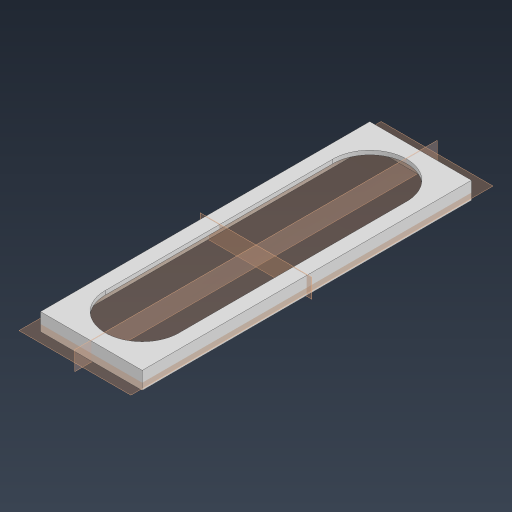
# Autodesk Inventor part: Крышка_крепления_динамика
Saved by Autodesk Inventor 2023.2 (Build 272271030, 271C)
## iProperties
Created: 2025-09-17
Part Number: Крышка_крепления_динамика
Material: Типовые
Document SubType Name: Modeling
Designer: Олег Коноваленко
Density: 1 g/cm^3
Appearance: По умолчанию
Author: Олег Коноваленко
Autodesk Inventor part; units mm, degrees
sketch "Эскиз1" plane through (0, 0, 0) normal (0, 1, 0) x (-1, 0, 0)
  line L0 (35, 120) -> (-35, 120)
  line L1 (-35, 120) -> (-35, -120)
  line L2 (-35, -120) -> (35, -120)
  line L3 (35, -120) -> (35, 120)
  line L4 (35, 120) -> (-35, -120) construction
  line L5 (-35, 120) -> (35, -120) construction
  point P0 (0, 0)
  dimension "d0" = 70
  dimension "d1" = 240
  constraints: 12 end point, 2 midpoint, 2 parallel, 1 horizontal, 1 perpendicular
  measures "d0" distance of L1.end L2.end
  measures "d1" distance of L2.end L0.start
extrude "Выдавливание1" add sketch "Эскиз1" along normal mid plane 10
shell "Оболочка1" thickness 3 outward yes removed faces 1 at (-11.6667, -5, -40)
sketch "Эскиз2" plane through (0, 8, 0) normal (0, 1, 0) x (1, 0, 0)
  line L0 (0, 85) -> (0, -85) construction
  line L1 (-27.5, 85) -> (-27.5, -85)
  line L2 (27.5, -85) -> (27.5, 85)
  arc A0 (27.5, 85) -> (-27.5, 85) centre (0, 85) ccw
  arc A1 (-27.5, -85) -> (27.5, -85) centre (0, -85) ccw
  point P0 (0, 0)
  point P1 (0, -112.5)
  point P2 (0, 112.5)
  dimension "d5" = 225
  dimension "d6" = 55
  constraints: 8 end point, 6 point on circle, 4 tangent, 2 centre point, 1 midpoint, 1 parallel, 1 vertical
  measures "d5" distance of point (0, -112.5) point (0, 112.5)
  measures "d6" distance between parallel lines of L1 L2
extrude "Выдавливание2" cut sketch "Эскиз2" against normal up to next
